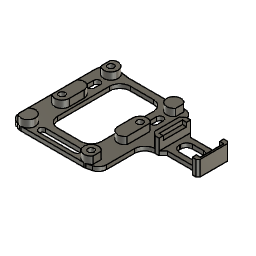
LM2596_mount_double v5 (Autodesk Fusion 360 design; units mm, degrees)
Autodesk Fusion 360 part; units mm, degrees
note: some values were not read from the file. Set by a fixed rule: which sketch regions a step uses.
sketch "board size and holes" plane through (0, 0, 0) normal (0, 0, 1) x (1, 0, 0)
  line L0 (0, 0) -> (43.1, 0)
  line L1 (43.1, 0) -> (43.1, 21.3)
  line L2 (43.1, 21.3) -> (0, 21.3)
  line L3 (0, 21.3) -> (0, 0)
  circle A0 centre (6, 18.55) radius 3.5
  circle A1 centre (6, 2.05) radius 3.5
  circle A2 centre (36.7, 2.05) radius 3.5
  circle A3 centre (36.7, 18.55) radius 3.5
  circle A4 centre (36.7, 2.05) radius 1.5
  circle A5 centre (6, 18.55) radius 1.5
  line L4 (0, 45.1) -> (0, 23.8)
  circle A6 centre (6, 42.35) radius 3.5
  circle A7 centre (6, 42.35) radius 1.5
  circle A8 centre (6, 25.85) radius 3.5
  line L5 (0, 23.8) -> (43.1, 23.8)
  circle A9 centre (36.7, 25.85) radius 3.5
  circle A10 centre (36.7, 25.85) radius 1.5
  circle A11 centre (36.7, 42.35) radius 3.5
  line L6 (43.1, 23.8) -> (43.1, 45.1)
  line L7 (43.1, 45.1) -> (0, 45.1)
  line L8 (43.1, 21.3) -> (43.1, 26.3)
  line L9 (0, 21.3) -> (0, 26.3)
  point P0 (6, 17.05)
  point P1 (36.7, 3.55)
  point P2 (7.5, 18.55)
  point P3 (35.2, 2.05)
  dimension "d7" = 43.1
  dimension "d8" = 21.3
  dimension "d14" = 3
  dimension "d15" = 3
  dimension "d25" = 4.25
  dimension "d26" = 3.55
  dimension "d27" = 2
  dimension "d38" = 7.9
  dimension "d39" = 7.5
  dimension "d46" = 2.5
  dimension "d47" = 23.8
  constraint horizontal L0
  constraint vertical L1
  constraint horizontal L2
  constraint vertical L3
  constraint coincident L0.start L3.end
  constraint horizontal A1.centre A2.centre
  constraint vertical A0.centre A1.centre
  constraint vertical A2.centre A3.centre
  constraint horizontal A0.centre A3.centre
  constraint equal A0 A3
  constraint equal A2 A3
  constraint equal A1 A2
  constraint concentric A2 A4
  constraint concentric A0 A5
  constraint coincident A5 P0
  constraint coincident A4 P1
  constraint vertical A0.centre P0
  constraint vertical A2.centre P1
  constraint coincident A5 P2
  constraint coincident A4 P3
  constraint horizontal A0.centre P2
  constraint horizontal A2.centre P3
  measures "d7" distance of L1.end L2.end
  measures "d8" distance of L0.end L1.end
  measures "d14" diameter of A5
  measures "d15" diameter of A4
  measures "d25" distance of L2 P0
  measures "d26" distance of L0 P1
  measures "d27" distance of A0 A5
  measures "d38" distance of L1 P3
  measures "d39" distance of L3 P2
extrude "Extrude5" add sketch "board size and holes" along normal blind 2 makes body 1
extrude "Extrude6" add sketch "board size and holes" along normal blind 3.5 from surface at 2 contours L0 A1 | L0 A1 | L2 A0 | L2 A0 | L0 A2 | L0 A2 | A8 L5 | A8 L5 | L2 A3 | L2 A3 | A6 L7 | A6 L7 | L5 A9 | L5 A9 | A11 L7 | A11 L7 bodies 1
sketch "Sketch3" plane through (0, 0, 2) normal (0, 0, 1) x (-1, 0, 0)
  circle A0 centre (-36.7, -18.55) radius 3.5
  circle A1 centre (-6, -25.85) radius 3.5
  circle A2 centre (-6, -18.55) radius 3.5
  circle A3 centre (-36.7, -25.85) radius 3.5
  arc A4 (-39.5368, 0) -> (-33.8632, 0) centre (-36.7, -2.05) ccw
  line L0 (-39.5368, 0) -> (-43.1, 0)
  line L1 (-43.1, 0) -> (-43.1, -45.1)
  line L2 (-43.1, -45.1) -> (-38.8651, -45.1)
  arc A5 (-34.5349, -45.1) -> (-38.8651, -45.1) centre (-36.7, -42.35) ccw
  line L3 (-34.5349, -45.1) -> (-8.1651, -45.1)
  arc A6 (-3.8349, -45.1) -> (-8.1651, -45.1) centre (-6, -42.35) ccw
  line L4 (-3.8349, -45.1) -> (0, -45.1)
  line L5 (0, -45.1) -> (0, 0)
  line L6 (0, 0) -> (-3.1632, 0)
  arc A7 (-8.8368, 0) -> (-3.1632, 0) centre (-6, -2.05) ccw
  line L7 (-8.8368, 0) -> (-33.8632, 0)
  line L8 (-6, -35.55) -> (-6, -32.65) construction
  line L9 (-29.9, -2.05) -> (-12.8, -2.05) construction
  line L10 (-36.7, -32.65) -> (-36.7, -35.55) construction
  line L11 (-4.3, -35.55) -> (-4.3, -32.65)
  arc A8 (-4.3, -32.65) -> (-7.7, -32.65) centre (-6, -32.65) ccw
  line L12 (-7.7, -32.65) -> (-7.7, -35.55)
  arc A9 (-7.7, -35.55) -> (-4.3, -35.55) centre (-6, -35.55) ccw
  line L13 (-6, -35.55) -> (-6, -32.65) construction
  line L14 (-35, -35.55) -> (-35, -32.65)
  arc A10 (-35, -32.65) -> (-38.4, -32.65) centre (-36.7, -32.65) ccw
  line L15 (-38.4, -32.65) -> (-38.4, -35.55)
  arc A11 (-38.4, -35.55) -> (-35, -35.55) centre (-36.7, -35.55) ccw
  line L16 (-36.7, -35.55) -> (-36.7, -32.65) construction
  line L17 (-29.9, -3.75) -> (-12.8, -3.75)
  arc A12 (-12.8, -3.75) -> (-12.8, -0.35) centre (-12.8, -2.05) ccw
  line L18 (-12.8, -0.35) -> (-29.9, -0.35)
  arc A13 (-29.9, -0.35) -> (-29.9, -3.75) centre (-29.9, -2.05) ccw
  line L19 (-29.9, -2.05) -> (-12.8, -2.05) construction
  line L20 (-6, -35.55) -> (-6, -42.35) construction
  line L21 (-6, -32.65) -> (-6, -25.85) construction
  line L22 (-6, -2.05) -> (-12.8, -2.05) construction
  line L23 (-29.9, -2.05) -> (-36.7, -2.05) construction
  point P0 (-6, -37.25)
  point P1 (-6, -38.85)
  point P2 (-11.1, -2.05)
  point P3 (-9.5, -2.05)
  dimension "d57" = 1.7
  dimension "d58" = 1.6
  dimension "d59" = 1.6
  constraint parallel L1 L8
  constraint perpendicular L1 L9
  constraint vertical L10
  constraint vertical A6.centre L8.start
  constraint vertical A3.centre L10.start
  constraint horizontal A4.centre L9.start
  constraint tangent L11 A8
  constraint tangent A8 L12
  constraint parallel L11 L12
  constraint tangent L12 A9
  constraint tangent L11 A9
  constraint coincident L8.end A8.centre
  constraint parallel L8 L13
  constraint coincident L8.start A9.centre
  constraint tangent L14 A10
  constraint tangent A10 L15
  constraint parallel L14 L15
  constraint tangent L15 A11
  constraint tangent L14 A11
  constraint coincident L10.start A10.centre
  constraint parallel L10 L16
  constraint coincident L10.end A11.centre
  constraint tangent L17 A12
  constraint tangent A12 L18
  constraint parallel L17 L18
  constraint tangent L18 A13
  constraint tangent L17 A13
  constraint coincident L9.end A12.centre
  constraint perpendicular L10 L19
  constraint coincident L9.start A13.centre
  constraint equal A9 A11
  constraint equal A11 A12
  constraint equal L12 L14
  constraint coincident A6.centre L20.end
  constraint coincident A1.centre L21.end
  constraint coincident A7.centre L22.start
  constraint coincident A4.centre L23.end
  constraint equal L20 L21
  constraint equal L22 L23
  constraint horizontal L8.start L10.end
  constraint midpoint A9 P0
  constraint midpoint A6 P1
  constraint midpoint A12 P2
  constraint coincident L22 P3
  constraint coincident A7 P3
  measures "d57" radius of A9
  measures "d58" distance of P0 P1
  measures "d59" distance of P2 P3
extrude "Extrude7" cut sketch "Sketch3" against normal up to surface (2 mm away) contours L11 A8 L12 A9 | L14 A10 L15 A11 | L17 A12 L18 A13 bodies 1
sketch "Sketch4" plane through (0, 0, 2) normal (0, 0, 1) x (-1, 0, 0)
  arc A0 (-29.9, -0.35) -> (-29.9, -3.75) centre (-29.9, -2.05) ccw
  line L0 (-29.9, -0.35) -> (-12.8, -0.35)
  arc A1 (-12.8, -3.75) -> (-12.8, -0.35) centre (-12.8, -2.05) ccw
  line L1 (-12.8, -3.75) -> (-29.9, -3.75)
  arc A2 (-7.7, -35.55) -> (-4.3, -35.55) centre (-6, -35.55) ccw
  line L2 (-7.7, -35.55) -> (-7.7, -32.65)
  arc A3 (-4.3, -32.65) -> (-7.7, -32.65) centre (-6, -32.65) ccw
  line L3 (-4.3, -32.65) -> (-4.3, -35.55)
  arc A4 (-38.4, -35.55) -> (-35, -35.55) centre (-36.7, -35.55) ccw
  line L4 (-38.4, -35.55) -> (-38.4, -32.65)
  arc A5 (-35, -32.65) -> (-38.4, -32.65) centre (-36.7, -32.65) ccw
  line L5 (-35, -32.65) -> (-35, -35.55)
  circle A6 centre (-36.7, -18.55) radius 3.5
  circle A7 centre (-6, -25.85) radius 3.5
  circle A8 centre (-6, -18.55) radius 3.5
  circle A9 centre (-36.7, -25.85) radius 3.5
  arc A10 (-39.5368, 0) -> (-33.8632, 0) centre (-36.7, -2.05) ccw
  line L6 (-39.5368, 0) -> (-43.1, 0)
  line L7 (-43.1, 0) -> (-43.1, -45.1)
  line L8 (-43.1, -45.1) -> (-38.8651, -45.1)
  arc A11 (-34.5349, -45.1) -> (-38.8651, -45.1) centre (-36.7, -42.35) ccw
  line L9 (-34.5349, -45.1) -> (-8.1651, -45.1)
  arc A12 (-3.8349, -45.1) -> (-8.1651, -45.1) centre (-6, -42.35) ccw
  line L10 (-3.8349, -45.1) -> (0, -45.1)
  line L11 (0, -45.1) -> (0, 0)
  line L12 (0, 0) -> (-3.1632, 0)
  arc A13 (-8.8368, 0) -> (-3.1632, 0) centre (-6, -2.05) ccw
  line L13 (-8.8368, 0) -> (-33.8632, 0)
  line L14 (-10.7, -42.1) -> (-32, -42.1)
  line L15 (-32, -42.1) -> (-32, -6.75)
  line L16 (-32, -6.75) -> (-10.7, -6.75)
  line L17 (-10.7, -6.75) -> (-10.7, -42.1)
  dimension "d63" = 3
  dimension "d64" = 3
  dimension "d65" = 3
  dimension "d66" = 3
  constraint horizontal L14
  constraint vertical L15
  constraint horizontal L16
  constraint vertical L17
  measures "d63" distance of L2 L17
  measures "d64" distance of L5 L15
  measures "d65" distance of L1 L16
  measures "d66" distance of L9 L14
extrude "Extrude8" cut sketch "Sketch4" against normal up to surface (2 mm away) contours L14 L15 L16 L17 bodies 1
sketch "Sketch5" plane through (0, 0, 2) normal (0, 0, 1) x (-1, 0, 0)
  line L0 (-32, -6.75) -> (-10.7, -6.75)
  line L1 (-10.7, -6.75) -> (-10.7, -42.1)
  line L2 (-10.7, -42.1) -> (-32, -42.1)
  line L3 (-32, -42.1) -> (-32, -6.75)
  arc A0 (-29.9, -0.35) -> (-29.9, -3.75) centre (-29.9, -2.05) ccw
  line L4 (-29.9, -0.35) -> (-12.8, -0.35)
  arc A1 (-12.8, -3.75) -> (-12.8, -0.35) centre (-12.8, -2.05) ccw
  line L5 (-12.8, -3.75) -> (-29.9, -3.75)
  arc A2 (-7.7, -35.55) -> (-4.3, -35.55) centre (-6, -35.55) ccw
  line L6 (-7.7, -35.55) -> (-7.7, -32.65)
  arc A3 (-4.3, -32.65) -> (-7.7, -32.65) centre (-6, -32.65) ccw
  line L7 (-4.3, -32.65) -> (-4.3, -35.55)
  arc A4 (-38.4, -35.55) -> (-35, -35.55) centre (-36.7, -35.55) ccw
  line L8 (-38.4, -35.55) -> (-38.4, -32.65)
  arc A5 (-35, -32.65) -> (-38.4, -32.65) centre (-36.7, -32.65) ccw
  line L9 (-35, -32.65) -> (-35, -35.55)
  circle A6 centre (-36.7, -18.55) radius 3.5
  circle A7 centre (-6, -25.85) radius 3.5
  circle A8 centre (-6, -18.55) radius 3.5
  circle A9 centre (-36.7, -25.85) radius 3.5
  arc A10 (-39.5368, 0) -> (-33.8632, 0) centre (-36.7, -2.05) ccw
  line L10 (-39.5368, 0) -> (-43.1, 0)
  line L11 (-43.1, 0) -> (-43.1, -45.1)
  line L12 (-43.1, -45.1) -> (-38.8651, -45.1)
  arc A11 (-34.5349, -45.1) -> (-38.8651, -45.1) centre (-36.7, -42.35) ccw
  line L13 (-34.5349, -45.1) -> (-8.1651, -45.1)
  arc A12 (-3.8349, -45.1) -> (-8.1651, -45.1) centre (-6, -42.35) ccw
  line L14 (-3.8349, -45.1) -> (0, -45.1)
  line L15 (0, -45.1) -> (0, 0)
  line L16 (0, 0) -> (-3.1632, 0)
  arc A13 (-8.8368, 0) -> (-3.1632, 0) centre (-6, -2.05) ccw
  line L17 (-8.8368, 0) -> (-33.8632, 0)
  line L18 (-6, 1.45) -> (-36.7, 1.45)
  circle A14 centre (-36.7, -2.05) radius 3.5
  circle A15 centre (-6, -2.05) radius 3.5
  line L19 (-5.1153, 1.3364) -> (0, 0)
  line L20 (-43.1, 0) -> (-37.5245, 1.3515)
  line L21 (-43.1, -45.1) -> (-37.1211, -45.8246)
  line L22 (-30.3, -45.1) -> (-36.2789, -45.8246)
  line L23 (0, -45.1) -> (-5.5491, -45.8208)
  line L24 (-12, -45.1) -> (-6.4509, -45.8208)
  circle A16 centre (-6, -42.35) radius 3.5
  circle A17 centre (-36.7, -42.35) radius 3.5
  constraint horizontal L18
  constraint coincident L18.end A14
  constraint coincident L18.start A15
  constraint tangent L18 A15
  constraint coincident A15 L19.start
  constraint coincident L15.end L16.start
  constraint coincident L10.end L11.start
  constraint coincident A14 L20.end
  constraint tangent A14 L20
  constraint tangent A15 L19
  constraint coincident L11.end L12.start
  constraint coincident L13 L22.start
  constraint coincident L14.end L15.start
  constraint coincident L13 L24.start
  constraint tangent L23 A16
  constraint tangent L24 A16
  constraint tangent L22 A17
  constraint tangent L21 A17
  constraint coincident L21.end A17
  constraint coincident L22.end A17
  constraint coincident L24.end A16
  constraint coincident L23.end A16
  constraint equal L23 L24
  constraint equal L21 L22
extrude "Extrude9" add sketch "Sketch5" against normal up to surface (2 mm away) contours L10 A14 L20 | L17 L18 A14 A15 | L12 L21 A17 | L13 L22 A17 | L16 A15 L19 | L13 L24 A16 | L14 L23 A16 bodies 1
fillet "Fillet1" radius 5 4 edges at (10.7, 42.1, 1) (32, 42.1, 1) (32, 6.75, 1) (10.7, 6.75, 1) on bodies 1
fillet "Fillet2" radius 5 2 edges at (0, 0, 1) (0, 45.1, 1) on bodies 1
sketch "Sketch6" plane through (0, 0, 0) normal (0, 0, 1) x (1, 0, 0)
  line L0 (48.1, 35.16) -> (68.22, 35.16)
  line L1 (68.22, 35.16) -> (68.22, 23.8)
  line L2 (68.22, 23.8) -> (48.1, 23.8)
  line L3 (48.1, 23.8) -> (48.1, 35.16)
  line L4 (43.1, 0) -> (43.1, 45.1) construction
  line L5 (0, 23.8) -> (43.1, 23.8) construction
  dimension "d80" = 11.36
  dimension "d81" = 20.12
  dimension "d83" = 5
  constraint horizontal L0
  constraint vertical L1
  constraint horizontal L2
  constraint vertical L3
  constraint horizontal L2.end L5.end
  measures "d80" distance of L0.end L1.end
  measures "d81" distance of L1.end L2.end
  measures "d83" distance of L3 L4
extrude "Extrude10" add sketch "Sketch6" along normal blind 2 separate body makes body 2
sketch "Sketch7" plane through (0, 0, 2) normal (0, 0, 1) x (-1, 0, 0)
  line L0 (-48.1, -23.8) -> (-68.22, -23.8)
  line L1 (-68.22, -23.8) -> (-68.22, -35.16)
  line L2 (-68.22, -35.16) -> (-48.1, -35.16)
  line L3 (-48.1, -35.16) -> (-48.1, -23.8)
  line L4 (-50.1, -35.16) -> (-50.1, -23.8)
  line L5 (-66.22, -23.8) -> (-66.22, -35.16)
  dimension "d86" = 2
  dimension "d87" = 2
  constraint coincident L2 L4.start
  constraint coincident L0 L4.end
  constraint perpendicular L0 L4
  constraint coincident L0 L5.start
  constraint coincident L2 L5.end
  constraint perpendicular L2 L5
  measures "d86" distance of L3 L4
  measures "d87" distance of L1 L5
extrude "Extrude11" add sketch "Sketch7" along normal blind 3.5 contours L0 L2 L3 L4 | L0 L1 L2 L5 bodies 2
sketch "Sketch9" plane through (0, 0, 0) normal (0, 0, 1) x (1, 0, 0)
  line L0 (48.1, 35.16) -> (46.1, 35.16)
  line L1 (46.1, 35.16) -> (46.1, 23.8)
  line L2 (46.1, 23.8) -> (48.1, 23.8)
  line L3 (48.1, 23.8) -> (48.1, 35.16)
  line L4 (68.22, 35.16) -> (70.22, 35.16)
  line L5 (70.22, 35.16) -> (70.22, 23.8)
  line L6 (70.22, 23.8) -> (68.22, 23.8)
  line L7 (68.22, 23.8) -> (68.22, 35.16)
  line L8 (48.1, 23.8) -> (50.1, 23.8)
  line L9 (50.1, 35.16) -> (48.1, 35.16)
  line L10 (68.22, 35.16) -> (66.22, 35.16)
  line L11 (48.1, 35.16) -> (48.1, 23.8)
  line L12 (68.22, 23.8) -> (68.22, 35.16)
  line L13 (48.1, 35.16) -> (50.1, 35.16)
  line L14 (50.1, 35.16) -> (50.1, 37.16)
  line L15 (50.1, 37.16) -> (46.1, 37.16)
  line L16 (46.1, 37.16) -> (46.1, 35.16)
  line L17 (48.1, 23.8) -> (50.1, 23.8)
  line L18 (50.1, 23.8) -> (50.1, 21.8)
  line L19 (50.1, 21.8) -> (46.1, 21.8)
  line L20 (46.1, 21.8) -> (46.1, 23.8)
  line L21 (50.1, 23.8) -> (50.1, 35.16)
  line L22 (58.16, 35.16) -> (58.16, 23.8) construction
  line L23 (66.22, 35.16) -> (50.1, 35.16) construction
  line L24 (50.1, 23.8) -> (66.22, 23.8) construction
  line L25 (66.22, 37.16) -> (70.22, 37.16)
  line L26 (70.22, 37.16) -> (70.22, 35.16)
  line L27 (66.22, 35.16) -> (66.22, 37.16)
  line L28 (66.22, 23.8) -> (66.22, 21.8)
  line L29 (70.22, 21.8) -> (70.22, 23.8)
  line L30 (66.22, 21.8) -> (70.22, 21.8)
  line L31 (70.22, 35.16) -> (66.22, 35.16)
  line L32 (70.22, 23.8) -> (66.22, 23.8)
  dimension "d90" = 2
  dimension "d91" = 2
  constraint horizontal L0
  constraint vertical L1
  constraint horizontal L2
  constraint vertical L3
  constraint horizontal L4
  constraint vertical L5
  constraint horizontal L6
  constraint vertical L7
  constraint collinear L2 L8
  constraint collinear L2 L6
  constraint collinear L0 L9
  constraint collinear L4 L10
  constraint collinear L3 L11
  constraint collinear L7 L12
  constraint equal L0 L4
  constraint horizontal L13
  constraint vertical L14
  constraint horizontal L15
  constraint vertical L16
  constraint horizontal L17
  constraint vertical L18
  constraint horizontal L19
  constraint vertical L20
  constraint collinear L14 L21
  constraint collinear L18 L21
  constraint vertical L22
  constraint midpoint L22.start L23
  constraint midpoint L22.end L24
  constraint equal L14 L18
  constraint symmetric L0.end L22 L4.end
  constraint symmetric L1.end L22 L5.end
  constraint symmetric L9.start L22 L10.end
  constraint symmetric L14.end L22 L25.start
  constraint symmetric L15.end L22 L25.end
  constraint symmetric L8.end L22 L24.end
  constraint symmetric L18.end L22 L28.end
  constraint symmetric L19.end L22 L29.start
  measures "d90" distance of L0.start L0.end
  measures "d91" distance of L9.start L14.end
extrude "Extrude12" add sketch "Sketch9" along normal up to surface (7.42 mm away) contours L0 L1 L2 L3 L11 | L0 L9 L13 L14 L15 L16 | L2 L8 L17 L18 L19 L20 | L4 L10 L25 L26 L27 L31 | L4 L5 L6 L7 L12 L31 L32 | L6 L28 L29 L30 L32 bodies 2
sketch "Sketch10" plane through (0, 0, 2) normal (0, 0, 1) x (-1, 0, 0)
  line L0 (-27, -6.75) -> (-15.7, -6.75)
  arc A0 (-10.7, -11.75) -> (-15.7, -6.75) centre (-15.7, -11.75) ccw
  line L1 (-10.7, -11.75) -> (-10.7, -37.1)
  arc A1 (-15.7, -42.1) -> (-10.7, -37.1) centre (-15.7, -37.1) ccw
  line L2 (-15.7, -42.1) -> (-27, -42.1)
  arc A2 (-32, -37.1) -> (-27, -42.1) centre (-27, -37.1) ccw
  line L3 (-32, -37.1) -> (-32, -11.75)
  arc A3 (-27, -6.75) -> (-32, -11.75) centre (-27, -11.75) ccw
  arc A4 (-29.9, -0.35) -> (-29.9, -3.75) centre (-29.9, -2.05) ccw
  line L4 (-29.9, -0.35) -> (-12.8, -0.35)
  arc A5 (-12.8, -3.75) -> (-12.8, -0.35) centre (-12.8, -2.05) ccw
  line L5 (-12.8, -3.75) -> (-29.9, -3.75)
  arc A6 (-7.7, -35.55) -> (-4.3, -35.55) centre (-6, -35.55) ccw
  line L6 (-7.7, -35.55) -> (-7.7, -32.65)
  arc A7 (-4.3, -32.65) -> (-7.7, -32.65) centre (-6, -32.65) ccw
  line L7 (-4.3, -32.65) -> (-4.3, -35.55)
  arc A8 (-38.4, -35.55) -> (-35, -35.55) centre (-36.7, -35.55) ccw
  line L8 (-38.4, -35.55) -> (-38.4, -32.65)
  arc A9 (-35, -32.65) -> (-38.4, -32.65) centre (-36.7, -32.65) ccw
  line L9 (-35, -32.65) -> (-35, -35.55)
  circle A10 centre (-36.7, -18.55) radius 3.5
  circle A11 centre (-6, -25.85) radius 3.5
  circle A12 centre (-6, -18.55) radius 3.5
  circle A13 centre (-36.7, -25.85) radius 3.5
  arc A14 (-4.3559, -45.6658) -> (0, -40.7075) centre (-5, -40.7075) ccw
  line L10 (0, -40.7075) -> (0, -3.8616)
  arc A15 (0, -3.8616) -> (-3.7362, 0.9761) centre (-5, -3.8616) ccw
  line L11 (-3.7362, 0.9761) -> (-5.1153, 1.3364)
  arc A16 (-6, 1.45) -> (-5.1153, 1.3364) centre (-6, -2.05) ccw
  line L12 (-6, 1.45) -> (-36.7, 1.45)
  arc A17 (-37.5245, 1.3515) -> (-36.7, 1.45) centre (-36.7, -2.05) ccw
  line L13 (-37.5245, 1.3515) -> (-43.1, 0)
  line L14 (-43.1, 0) -> (-43.1, -45.1)
  line L15 (-43.1, -45.1) -> (-37.1211, -45.8246)
  arc A18 (-36.2789, -45.8246) -> (-37.1211, -45.8246) centre (-36.7, -42.35) ccw
  line L16 (-36.2789, -45.8246) -> (-30.3, -45.1)
  line L17 (-30.3, -45.1) -> (-12, -45.1)
  line L18 (-12, -45.1) -> (-6.4509, -45.8208)
  arc A19 (-5.5491, -45.8208) -> (-6.4509, -45.8208) centre (-6, -42.35) ccw
  line L19 (-5.5491, -45.8208) -> (-4.3559, -45.6658)
  line L20 (-43.1, -21.8) -> (-46.1, -21.8)
  line L21 (-43.1, -37.16) -> (-46.1, -37.16)
  line L22 (-46.1, -21.8) -> (-46.1, -37.16)
  point P0 (-46.1, -37.16)
  point P1 (-46.1, -21.8)
  constraint coincident L14 L20.start
  constraint perpendicular L14 L20
  constraint coincident L14 L21.start
  constraint coincident P0 L21.end
  constraint coincident P1 L20.end
  constraint horizontal L21
extrude "Extrude13" add sketch "Sketch10" against normal up to surface (2 mm away) contours L14 L20 L21 L22 bodies 1 2
fillet "Fillet3" radius 5 2 edges at (43.1, 21.8, 1) (43.1, 37.16, 1) on bodies 1
chamfer "Chamfer1" distance 2 angle 45 4 edges at (50.1, 23.8, 1) (50.1, 35.16, 1) (66.22, 23.8, 1) (66.22, 35.16, 1) on bodies 1
sketch "Sketch11" plane through (0, 0, 5.5) normal (0, 0, 1) x (-1, 0, 0)
  circle A0 centre (-6, -25.85) radius 3.5
  line L0 (-2.5, -25.85) -> (-2.5, -18.55)
  line L1 (-9.5, -25.85) -> (-9.5, -18.5553)
  line L2 (-33.2, -25.85) -> (-33.2, -18.5578)
  line L3 (-40.2, -25.85) -> (-40.2, -18.542)
  circle A1 centre (-6, -18.55) radius 3.5
  circle A2 centre (-36.7, -25.85) radius 3.5
  circle A3 centre (-36.7, -18.55) radius 3.5
  constraint coincident A0 L0.start
  constraint vertical L0
  constraint coincident A0 L1.start
  constraint vertical L1
  constraint vertical L2
  constraint vertical L3
  constraint coincident L0.end A1
  constraint coincident L1.end A1
  constraint coincident L2.start A2
  constraint coincident L3.start A2
  constraint coincident L3.end A3
  constraint coincident L2.end A3
  constraint tangent A0 L0
  constraint tangent A0 L1
  constraint tangent L2 A2
  constraint tangent L3 A2
extrude "Extrude14" add sketch "Sketch11" against normal up to surface (3.5 mm away) contours A0 L0 L1 A1 | L2 L3 A2 A3 bodies 1
sketch "Sketch12" plane through (0, 0, 5.5) normal (0, 0, 1) x (-1, 0, 0)
  circle A0 centre (-6, -18.55) radius 1.5
  arc A1 (-9.5, -25.85) -> (-2.5, -25.85) centre (-6, -25.85) ccw
  line L0 (-2.5, -25.85) -> (-2.5, -18.55)
  arc A2 (-2.5, -18.55) -> (-9.5, -18.5553) centre (-6, -18.55) ccw
  line L1 (-9.5, -18.5553) -> (-9.5, -25.85)
  line L2 (0, -45.8208) -> (-3.5, -45.8208)
  line L3 (-3.5, -45.8208) -> (-3.5, 1.3364)
  line L4 (-3.5, 1.3364) -> (0, 1.3364)
  line L5 (0, 1.3364) -> (0, -45.8208)
  line L6 (0, -40.7075) -> (0, -3.8616)
  line L7 (-39.6, -45.8246) -> (-43.1, -45.8246)
  line L8 (-43.1, -45.8246) -> (-43.1, 1.3515)
  line L9 (-43.1, 1.3515) -> (-39.6, 1.3515)
  line L10 (-39.6, 1.3515) -> (-39.6, -45.8246)
  line L11 (-43.1, 0) -> (-43.1, -16.8)
  point P0 (-5.5491, -45.8208)
  point P1 (-5.1153, 1.3364)
  point P2 (-37.1211, -45.8246)
  point P3 (-37.5245, 1.3515)
  dimension "d102" = 3.5
  dimension "d103" = 3.5
  constraint horizontal L2
  constraint vertical L3
  constraint horizontal L4
  constraint vertical L5
  constraint collinear L5 L6
  constraint horizontal L2.end P0
  constraint horizontal L3.end P1
  constraint horizontal L7
  constraint vertical L8
  constraint horizontal L9
  constraint vertical L10
  constraint collinear L8 L11
  constraint horizontal L7.start P2
  constraint horizontal L9.end P3
  measures "d102" distance of L2.start L2.end
  measures "d103" distance of L7.start L7.end
extrude "Extrude15" cut sketch "Sketch12" against normal up to surface (3.5 mm away) contours A1 L0 A2 L3 | A1 L0 A2 L2 L3 L4 L5 L6 | L7 L8 L9 L10 L11 bodies 1
sketch "Sketch13" plane through (0, 0, 2) normal (0, 0, 1) x (-1, 0, 0)
  line L0 (-66.22, -21.8) -> (-66.22, -37.16)
  line L1 (-66.22, -37.16) -> (-64.22, -35.16)
  line L2 (-64.22, -35.16) -> (-52.1, -35.16)
  line L3 (-52.1, -35.16) -> (-50.1, -37.16)
  line L4 (-50.1, -37.16) -> (-50.1, -21.8)
  line L5 (-50.1, -21.8) -> (-52.1, -23.8)
  line L6 (-52.1, -23.8) -> (-64.22, -23.8)
  line L7 (-64.22, -23.8) -> (-66.22, -21.8)
  line L8 (-52.5, -32.76) -> (-63.82, -32.76)
  line L9 (-63.82, -32.76) -> (-63.82, -26.2)
  line L10 (-63.82, -26.2) -> (-52.5, -26.2)
  line L11 (-52.5, -26.2) -> (-52.5, -32.76)
  line L12 (-50.1, -23.8) -> (-50.1, -35.16)
  line L13 (-66.22, -35.16) -> (-66.22, -23.8)
  dimension "d106" = 2.4
  dimension "d107" = 2.4
  dimension "d108" = 2.4
  dimension "d109" = 2.4
  constraint horizontal L8
  constraint vertical L9
  constraint horizontal L10
  constraint vertical L11
  measures "d106" distance of L6 L10
  measures "d107" distance of L2 L8
  measures "d108" distance of L11 L12
  measures "d109" distance of L9 L13
extrude "Extrude16" cut sketch "Sketch13" against normal up to surface (2 mm away) contours L8 L9 L10 L11 bodies 1
fillet "Fillet4" radius 3 4 edges at (63.82, 32.76, 1) (52.5, 32.76, 1) (52.5, 26.2, 1) (63.82, 26.2, 1) on bodies 1
sketch "Sketch14" plane through (0, 0, 7.42) normal (0, 0, 1) x (-1, 0, 0)
  line L0 (-68.22, -23.8) -> (-66.22, -23.8)
  line L1 (-66.22, -23.8) -> (-66.22, -21.8)
  line L2 (-66.22, -21.8) -> (-70.22, -21.8)
  line L3 (-70.22, -21.8) -> (-70.22, -37.16)
  line L4 (-70.22, -37.16) -> (-66.22, -37.16)
  line L5 (-66.22, -37.16) -> (-66.22, -35.16)
  line L6 (-66.22, -35.16) -> (-68.22, -35.16)
  line L7 (-68.22, -35.16) -> (-68.22, -23.8)
  line L8 (-69.02, -37.16) -> (-69.02, -21.8)
  dimension "d114" = 1.2
  constraint coincident L4 L8.start
  constraint coincident L2 L8.end
  constraint perpendicular L2 L8
  measures "d114" distance of L3 L8
extrude "Extrude17" cut sketch "Sketch14" against normal blind 21 contours L2 L3 L4 L8 bodies 1
chamfer "Chamfer2" distance 1 angle 45 2 edges at (69.02, 21.8, 3.71) (69.02, 37.16, 3.71) on bodies 1
chamfer "Chamfer2" distance 2 angle 45 2 edges at (46.1, 21.3826, 4.71) (46.1, 37.5774, 4.71) on bodies 1
fillet "Fillet5" radius 4 2 edges at (43.1, 0, 1) (43.1, 45.1, 1) on bodies 1
extrude "Extrude1" [suppressed]
extrude "Extrude2" [suppressed]
equation "board_W = 21.3 mm" comment "tested"
equation "board_L = 43.1 mm" comment "tested"
equation "d7 = board_L"
equation "d8 = board_W"
equation "inHole_SpanL = 7.9 mm" comment "tested"
equation "outHole_SpanL = 7.5 mm" comment "tested"
equation "M3_D = 3 mm" comment "tested"
equation "d14 = M3_D"
equation "d15 = d14"
equation "inHole_SpanW = 3.55 mm" comment "tested"
equation "outHole_SpanW = 4.25 mm" comment "tested"
equation "d25 = outHole_SpanW"
equation "d26 = inHole_SpanW"
equation "d38 = inHole_SpanL"
equation "d39 = outHole_SpanL"
equation "interboard_d = 2.5 mm"
equation "d46 = interboard_d"
equation "d47 = interboard_d + board_W"
equation "standoff_H = 3.5 mm"
equation "bottom_t = 2 mm"
equation "bore_d = 1 mm"
equation "d51 = bottom_t"
equation "d54 = standoff_H"
equation "clearance = 0.2 mm"
equation "d57 = M3_D / 2 + clearance"
equation "d59 = d58"
equation "bore_D = 5.4 mm"
equation "d64 = d63"
equation "d65 = d63"
equation "d66 = d63"
equation "perfBoard_L = 20.12 mm"
equation "perfBoard_W = 11.36 mm"
equation "perfBoard_H = 1.52 mm"
equation "perfBoar_ledge = 2 mm"
equation "d80 = perfBoard_W"
equation "d81 = perfBoard_L"
equation "perfBoard_gap = 5 mm"
equation "d83 = perfBoard_gap"
equation "d84 = bottom_t"
equation "d86 = perfBoar_ledge"
equation "d87 = perfBoar_ledge"
equation "d88 = standoff_H"
equation "d90 = perfBoar_ledge"
equation "d91 = d90"
equation "d92 = perfBoard_H + clearance * 2"
equation "solder_clearance = 3.5 mm"
equation "d102 = solder_clearance"
equation "d103 = d102"
equation "d107 = d106"
equation "d108 = d106"
equation "d109 = d106"
